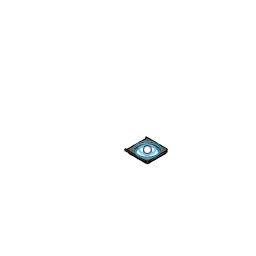
镜片罩 (Autodesk Fusion 360 design; units mm, degrees)
Autodesk Fusion 360 part; units mm, degrees
sketch "草图1" plane through (0, 0, 0) normal (0, 0, -1) x (1, 0, 0)
  arc A0 (2, -0.0127) -> (0.0127, -2) centre (2, -2) ccw
  line L0 (0.0127, -2) -> (0.0127, -24)
  arc A1 (0.0127, -24) -> (2, -25.9874) centre (2, -24) ccw
  line L1 (2, -25.9874) -> (98.0002, -25.9874)
  arc A2 (98.0002, -25.9874) -> (99.9875, -24) centre (98.0002, -24) ccw
  line L2 (99.9875, -24) -> (99.9875, -2)
  arc A3 (99.9875, -2) -> (98.0002, -0.0127) centre (98.0002, -2) ccw
  line L3 (98.0002, -0.0127) -> (2, -0.0127)
  line L4 (75.4874, -23.5) -> (75.4874, -2.5)
  arc A4 (76.5002, -1.4873) -> (75.4874, -2.5) centre (76.5002, -2.5) ccw
  line L5 (76.5002, -1.4873) -> (97.5002, -1.4873)
  arc A5 (98.5129, -2.5) -> (97.5002, -1.4873) centre (97.5002, -2.5) ccw
  line L6 (98.5129, -2.5) -> (98.5129, -23.5)
  arc A6 (97.5002, -24.5127) -> (98.5129, -23.5) centre (97.5002, -23.5) ccw
  line L7 (97.5002, -24.5127) -> (76.5002, -24.5127)
  arc A7 (75.4874, -23.5) -> (76.5002, -24.5127) centre (76.5002, -23.5) ccw
  circle A8 centre (70.0001, -13) radius 1
  circle A9 centre (49.3645, -3.302) radius 0.55
  circle A10 centre (46.8245, -3.302) radius 0.55
  circle A11 centre (44.2845, -3.302) radius 0.55
  circle A12 centre (41.7445, -3.302) radius 0.55
  circle A13 centre (16.6008, -2.667) radius 0.55
  circle A14 centre (14.0608, -2.667) radius 0.55
  circle A15 centre (2, -2) radius 1
  circle A16 centre (11.5207, -2.667) radius 0.55
  circle A17 centre (8.9807, -2.667) radius 0.55
  circle A18 centre (6.4407, -2.667) radius 0.55
  circle A19 centre (14.0778, -6.096) radius 0.55
  circle A20 centre (11.5378, -6.096) radius 0.55
  circle A21 centre (8.9978, -6.096) radius 0.55
  circle A22 centre (6.4578, -6.096) radius 0.55
  arc A23 (5.9253, -8.9448) -> (5.9253, -9.5448) centre (5.9253, -9.2448) ccw
  line L8 (5.9253, -8.9448) -> (7.1253, -8.9448)
  arc A24 (7.1253, -9.5448) -> (7.1253, -8.9448) centre (7.1253, -9.2448) ccw
  line L9 (7.1253, -9.5448) -> (5.9253, -9.5448)
  arc A25 (1.8754, -8.9448) -> (1.8754, -9.5448) centre (1.8754, -9.2448) ccw
  line L10 (1.8754, -8.9448) -> (2.7755, -8.9448)
  arc A26 (2.7755, -9.5448) -> (2.7755, -8.9448) centre (2.7755, -9.2448) ccw
  line L11 (2.7755, -9.5448) -> (1.8754, -9.5448)
  circle A27 centre (6.0255, -10.6796) radius 0.325
  arc A28 (67.9758, -20.2175) -> (68.5758, -20.2175) centre (68.2758, -20.2175) ccw
  line L12 (67.9758, -20.2175) -> (67.9758, -19.0175)
  arc A29 (68.5758, -19.0175) -> (67.9758, -19.0175) centre (68.2758, -19.0175) ccw
  line L13 (68.5758, -19.0175) -> (68.5758, -20.2175)
  circle A30 centre (66.8407, -20.1173) radius 0.325
  arc A31 (59.3258, -20.2175) -> (59.9258, -20.2175) centre (59.6258, -20.2175) ccw
  line L14 (59.3258, -20.2175) -> (59.3258, -19.0175)
  arc A32 (59.9258, -19.0175) -> (59.3258, -19.0175) centre (59.6258, -19.0175) ccw
  line L15 (59.9258, -19.0175) -> (59.9258, -20.2175)
  circle A33 centre (61.0606, -20.1173) radius 0.325
  arc A34 (67.9758, -24.2674) -> (68.5758, -24.2674) centre (68.2758, -24.2674) ccw
  line L16 (67.9758, -24.2674) -> (67.9758, -23.3674)
  arc A35 (68.5758, -23.3674) -> (67.9758, -23.3674) centre (68.2758, -23.3674) ccw
  line L17 (68.5758, -23.3674) -> (68.5758, -24.2674)
  arc A36 (59.3258, -24.2674) -> (59.9258, -24.2674) centre (59.6258, -24.2674) ccw
  line L18 (59.3258, -24.2674) -> (59.3258, -23.3674)
  arc A37 (59.9258, -23.3674) -> (59.3258, -23.3674) centre (59.6258, -23.3674) ccw
  line L19 (59.9258, -23.3674) -> (59.9258, -24.2674)
  circle A38 centre (6.0255, -16.4597) radius 0.325
  arc A39 (5.9253, -17.5948) -> (5.9253, -18.1948) centre (5.9253, -17.8948) ccw
  line L20 (5.9253, -17.5948) -> (7.1253, -17.5948)
  arc A40 (7.1253, -18.1948) -> (7.1253, -17.5948) centre (7.1253, -17.8948) ccw
  line L21 (7.1253, -18.1948) -> (5.9253, -18.1948)
  arc A41 (1.8754, -17.5948) -> (1.8754, -18.1948) centre (1.8754, -17.8948) ccw
  line L22 (1.8754, -17.5948) -> (2.7755, -17.5948)
  arc A42 (2.7755, -18.1948) -> (2.7755, -17.5948) centre (2.7755, -17.8948) ccw
  line L23 (2.7755, -18.1948) -> (1.8754, -18.1948)
  circle A43 centre (2, -24) radius 1
  line L24 (74.1113, -0.0127) -> (99.9875, -0.0127)
  line L25 (99.9875, -0.0127) -> (99.9875, -25.9874)
  line L26 (99.9875, -25.9874) -> (74.1113, -25.9874)
  line L27 (74.1113, -23.9874) -> (74.1113, -2.0127)
  arc A44 (74.1113, -2.0127) -> (72.1113, -0.0127) centre (72.1113, -2.0127) ccw
  arc A45 (72.1113, -25.9874) -> (74.1113, -23.9874) centre (72.1113, -23.9874) ccw
  dimension "d27" = 2
  dimension "d28" = 2
  constraint horizontal L24
  constraint vertical L25
  constraint horizontal L26
  constraint vertical L27
  constraint coincident L3 L24.start
  constraint coincident L24.start L27
  constraint tangent L27 A44
  constraint coincident L26.end L27
  constraint tangent L27 A45
  measures "d27" radius of A44
  measures "d28" radius of A45
extrude "拉伸1" add sketch "草图1" along normal up to surface (2 mm away) contours L1 A2 L2 A3 L3 L24 L25 L26 L27 A44 A45
sketch "草图2" plane through (0, 0, -2) normal (0, 0, -1) x (1, 0, 0)
  line L0 (76.1113, -25.9874) -> (98, -25.9874)
  line L1 (100, -23.9874) -> (100, -2)
  line L2 (98, 0) -> (76.1113, 0)
  line L3 (74.1113, -2) -> (74.1113, -23.9874)
  arc A0 (76.1113, 0) -> (74.1113, -2) centre (76.1113, -2) ccw
  arc A1 (74.1113, -23.9874) -> (76.1113, -25.9874) centre (76.1113, -23.9874) ccw
  arc A2 (100, -2) -> (98, 0) centre (98, -2) ccw
  arc A3 (98, -25.9874) -> (100, -23.9874) centre (98, -23.9874) ccw
  line L4 (75.1113, -2) -> (75.1113, -23.9874)
  arc A4 (75.1113, -23.9874) -> (76.1113, -24.9874) centre (76.1113, -23.9874) ccw
  line L5 (76.1113, -24.9874) -> (98, -24.9874)
  arc A5 (98, -24.9874) -> (99, -23.9874) centre (98, -23.9874) ccw
  line L6 (99, -23.9874) -> (99, -2)
  arc A6 (99, -2) -> (98, -1) centre (98, -2) ccw
  line L7 (98, -1) -> (76.1113, -1)
  arc A7 (76.1113, -1) -> (75.1113, -2) centre (76.1113, -2) ccw
  dimension "d31" = 2
  dimension "d32" = 2
  dimension "d33" = 2
  dimension "d34" = -1
  constraint horizontal L0
  constraint vertical L1
  constraint horizontal L2
  constraint vertical L3
  constraint tangent L2 A0
  constraint tangent L3 A0
  constraint tangent L0 A1
  constraint tangent L3 A1
  constraint equal A0 A1
  constraint tangent L1 A2
  constraint tangent L2 A2
  constraint tangent L0 A3
  constraint tangent L1 A3
  measures "d31" radius of A0
  measures "d32" radius of A2
  measures "d33" radius of A3
extrude "拉伸2" add sketch "草图2" along normal blind 1.5 contours L4 A4 L5 A5 L6 A6 L7 A7
fillet "圆角1" radius 0.9 tangency weight 1.15399 8 edges at (75.1113, 12.9937, -2) (75.4042, 1.2929, -2) (87.0556, 1, -2) (98.7071, 1.2929, -2) (99, 12.9937, -2) (98.7071, 24.6945, -2) (87.0556, 24.9874, -2) (75.4042, 24.6945, -2)
sketch "草图3" plane through (0, 0, -3.5) normal (0, 0, -1) x (1, 0, 0)
  arc A0 (76.1113, -1) -> (75.1113, -2) centre (76.1113, -2) ccw
  line L0 (75.1113, -2) -> (75.1113, -23.9874)
  arc A1 (75.1113, -23.9874) -> (76.1113, -24.9874) centre (76.1113, -23.9874) ccw
  line L1 (76.1113, -24.9874) -> (98, -24.9874)
  arc A2 (98, -24.9874) -> (99, -23.9874) centre (98, -23.9874) ccw
  line L2 (99, -23.9874) -> (99, -2)
  arc A3 (99, -2) -> (98, -1) centre (98, -2) ccw
  line L3 (98, -1) -> (76.1113, -1)
  circle A4 centre (87.0556, -12.9937) radius 7
  circle A5 centre (87.0556, -12.9937) radius 11.5
  dimension "d39" = 14
  dimension "d40" = 23
  constraint concentric A4 A5
  measures "d39" diameter of A4
  measures "d40" diameter of A5
extrude "拉伸3" cut sketch "草图3" against normal blind 4 contours A4
sketch "草图4" plane through (0, 0, -3.5) normal (0, 0, -1) x (1, 0, 0)
  circle A0 centre (87.0556, -12.9937) radius 7
  arc A1 (76.1113, -1) -> (75.1113, -2) centre (76.1113, -2) ccw
  line L0 (75.1113, -2) -> (75.1113, -23.9874)
  arc A2 (75.1113, -23.9874) -> (76.1113, -24.9874) centre (76.1113, -23.9874) ccw
  line L1 (76.1113, -24.9874) -> (98, -24.9874)
  arc A3 (98, -24.9874) -> (99, -23.9874) centre (98, -23.9874) ccw
  line L2 (99, -23.9874) -> (99, -2)
  arc A4 (99, -2) -> (98, -1) centre (98, -2) ccw
  line L3 (98, -1) -> (76.1113, -1)
  circle A5 centre (87.0556, -12.9937) radius 11.5
  circle A6 centre (87.0556, -12.9937) radius 8
  circle A7 centre (87.0556, -12.9937) radius 9
  dimension "d45" = 23
  dimension "d46" = 16
  dimension "d47" = 18
  constraint concentric A0 A5
  constraint concentric A5 A6
  constraint concentric A5 A7
  measures "d45" diameter of A5
  measures "d46" diameter of A6
  measures "d47" diameter of A7
extrude "拉伸4" add sketch "草图4" along normal blind 0.6 contours A6
sketch "草图5" plane through (0, 0, -3.5) normal (0, 0, -1) x (1, 0, 0)
  circle A0 centre (87.0556, -12.9937) radius 8
  arc A1 (76.1113, -1) -> (75.1113, -2) centre (76.1113, -2) ccw
  line L0 (75.1113, -2) -> (75.1113, -23.9874)
  arc A2 (75.1113, -23.9874) -> (76.1113, -24.9874) centre (76.1113, -23.9874) ccw
  line L1 (76.1113, -24.9874) -> (98, -24.9874)
  arc A3 (98, -24.9874) -> (99, -23.9874) centre (98, -23.9874) ccw
  line L2 (99, -23.9874) -> (99, -2)
  arc A4 (99, -2) -> (98, -1) centre (98, -2) ccw
  line L3 (98, -1) -> (76.1113, -1)
  circle A5 centre (87.0556, -12.9937) radius 11.25
  circle A6 centre (87.0556, -12.9937) radius 9.5
  dimension "d51" = 22.5
  dimension "d52" = 19
  constraint concentric A0 A5
  constraint concentric A5 A6
  measures "d51" diameter of A5
  measures "d52" diameter of A6
extrude "拉伸5" cut sketch "草图5" against normal blind 0.3 contours A5
sketch "草图6" plane through (0, 0, -2) normal (0, 0, 1) x (-1, 0, 0)
  circle A0 centre (-87.0556, -12.9937) radius 7
  line L0 (-98.5129, -2.5) -> (-98.5129, -23.5)
  arc A1 (-98.5129, -23.5) -> (-97.5002, -24.5127) centre (-97.5002, -23.5) ccw
  line L1 (-97.5002, -24.5127) -> (-76.5002, -24.5127)
  arc A2 (-76.5002, -24.5127) -> (-75.4874, -23.5) centre (-76.5002, -23.5) ccw
  line L2 (-75.4874, -23.5) -> (-75.4874, -2.5)
  arc A3 (-75.4874, -2.5) -> (-76.5002, -1.4873) centre (-76.5002, -2.5) ccw
  line L3 (-76.5002, -1.4873) -> (-97.5002, -1.4873)
  arc A4 (-97.5002, -1.4873) -> (-98.5129, -2.5) centre (-97.5002, -2.5) ccw
extrude "拉伸6" add sketch "草图6" along normal blind 2
sketch "草图7" plane through (0, 0, -3.5) normal (0, 0, -1) x (1, 0, 0)
  circle A0 centre (87.0556, -12.9937) radius 9.5
  circle A1 centre (87.0556, -12.9937) radius 8
  circle A2 centre (87.0556, -12.9937) radius 7
  dimension "d57" = 14
  constraint concentric A0 A2
  measures "d57" diameter of A2
extrude "拉伸7" add sketch "草图7" against normal blind 0.5 contours A2
sketch "草图8" plane through (0, 0, -3) normal (0, 0, 1) x (-1, 0, 0)
  circle A0 centre (-87.0556, -12.9937) radius 7
  circle A1 centre (-87.0556, -12.9937) radius 6.5
  dimension "d60" = 13
  constraint concentric A0 A1
  measures "d60" diameter of A1
extrude "拉伸8" cut sketch "草图8" against normal blind 5 contours A1
sketch "sketch 2307" plane through (0, 0, 0) normal (0, 0, 1) x (-1, 0, 0)
  circle A0 centre (-87.0556, -12.9937) radius 7
  circle A1 centre (-87.0556, -12.9937) radius 11.6
extrude "拉伸9" cut sketch "sketch 2307" against normal blind 2.5
sketch "sketch 2323" plane through (0, 0, -2.5) normal (0, 0, 1) x (-1, 0, 0)
  circle A0 centre (-87.0556, -12.9937) radius 10
extrude "拉伸10" cut sketch "sketch 2323" against normal blind 5
